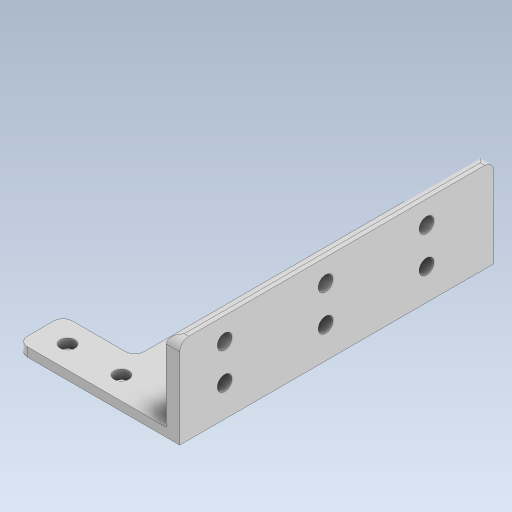
# Autodesk Inventor part: Holder Conveyor Kiri
Saved by Autodesk Inventor 2023.5 (Build 275446000, 446)
## iProperties
Created: 2025-10-12
Part Number: Holder Conveyor Kiri
Material: Generic
Document SubType Name: Modeling
Designer: Guntur
Density: 1 g/cm^3
Appearance: Default
Author: Guntur
## iProperties of the stored document Holder Conveyor Kiri_3DPrint.ipt
Created: 2025-10-20
Part Number: Holder Conveyor Kiri_3DPrint
Material: Generic
Document SubType Name: Modeling
Designer: Guntur
Density: 1 g/cm^3
Appearance: Default
Author: Guntur
Autodesk Inventor part; units mm, degrees
ref_plane "YZ Plane" through (0, 0, 0) normal (1, 0, 0) x (0, 1, 0)
ref_plane "XZ Plane" through (0, 0, 0) normal (0, 1, 0) x (-1, 0, 0)
ref_plane "XY Plane" through (0, 0, 0) normal (0, 0, 1) x (1, 0, 0)
sketch "Sketch1" plane through (0, 0, 0) normal (0, 1, 0) x (-1, 0, 0)
  circle A0 centre (0, 0) radius 1.65
  circle A1 centre (-12, 0) radius 1.65
  circle A2 centre (-20, -12.5) radius 1.65
  circle A3 centre (-20, -52.5) radius 1.65
  line L0 (-10, -30) -> (-30, -30)
  line L1 (-30, -30) -> (-30, 5)
  line L2 (-30, 5) -> (-10, 5)
  line L3 (-10, 5) -> (-10, -30)
  line L4 (-10, -30) -> (-30, 5) construction
  line L5 (-30, -30) -> (-10, 5) construction
  line L6 (-30, -5) -> (6, -5)
  line L7 (6, -5) -> (6, 5)
  line L8 (6, 5) -> (-30, 5)
  line L9 (-30, 5) -> (-30, -5)
  line L10 (-30, -5) -> (6, 5) construction
  line L11 (6, -5) -> (-30, 5) construction
  line L12 (-10, -30) -> (-30, -30)
  line L13 (-30, -30) -> (-30, -65)
  line L14 (-30, -65) -> (-10, -65)
  line L15 (-10, -65) -> (-10, -30)
  line L16 (-30, 5) -> (-27, 5)
  line L17 (-27, 5) -> (-27, -65)
  line L18 (-27, -65) -> (-30, -65)
  line L19 (-30, -65) -> (-30, 5)
  circle A4 centre (-20, -20) radius 1.65
  circle A5 centre (-20, -60) radius 1.65
  point P0 (-10, -5)
  dimension "d0" = 3.3
  dimension "d1" = 3.3
  dimension "d2" = 12
  dimension "d3" = 3.3
  dimension "d4" = 12.5
  dimension "d5" = 20
  dimension "d6" = 3.3
  dimension "d7" = 40
  dimension "d8" = 20
  dimension "d9" = 35
  dimension "d25" = 3.3
  dimension "d26" = 20
  dimension "d27" = 3.3
  dimension "d28" = 40
  constraints: 40 end point, 8 parallel, 6 centre point, 4 horizontal, 4 midpoint, 4 perpendicular, 2 point on line, 1 coincident
  measures "d0" diameter of A0
  measures "d1" diameter of A1
  measures "d2" distance of A1.centre point (0, 0)
  measures "d3" diameter of A2
  measures "d4" vertical distance of point (0, 0) A2.centre
  measures "d5" horizontal distance of point (0, 0) A2.centre
  measures "d6" diameter of A3
  measures "d7" distance of A2.centre A3.centre
  measures "d8" distance of L1.end L2.end
  measures "d9" distance of L13.end L12.end
  measures "d25" diameter of A4
  measures "d26" vertical distance of A1.centre A4.centre
  measures "d27" diameter of A5
  measures "d28" distance of A4.centre A5.centre
extrude "Extrusion1" add sketch "Sketch1" along normal blind 2 contours L15 L14 L17 L0 | L0 L17 L6 L3 | L6 L17 L2 L3 | L3 L8 L7 L6
extrude "Extrusion2" add sketch "Sketch1" along normal blind 20 contours L17 L14 L13 L0 | L0 L1 L6 L17 | L6 L1 L2 L17
sketch "Sketch2" plane through (30, 0, 5) normal (1, 0, 0) x (0, 0, -1)
  circle A0 centre (10, 15) radius 1.65
  line L0 (0, 0) -> (0, 20) projected
  circle A1 centre (55, 15) radius 1.65
  line L1 (70, 0) -> (70, 20) projected
  circle A2 centre (32.5, 15) radius 1.65
  line L2 (0, 20) -> (70, 20) projected
  line L3 (0, 2) -> (0, 20) projected
  line L4 (0, 11) -> (70, 11)
  circle A3 centre (10, 7) radius 1.65
  circle A4 centre (55, 7) radius 1.65
  circle A5 centre (32.5, 7) radius 1.65
  point P0 (5, 0)
  point P1 (70, 10)
  dimension "d14" = 3.3
  dimension "d15" = 10
  dimension "d16" = 3.3
  dimension "d18" = 3.3
  dimension "d21" = 5
  dimension "d22" = 5
  dimension "d23" = 5
  dimension "d24" = 15
  constraints: 6 centre point, 3 symmetric about line, 2 end point, 2 midpoint, 1 perpendicular, 1 point on line, 3 other
  measures "d14" diameter of A0
  measures "d15" distance from line of L0 A0.centre
  measures "d16" diameter of A1
  measures "d18" diameter of A2
  measures "d21" distance from line of L2 A0.centre
  measures "d22" distance from line of L2 A1.centre
  measures "d23" distance from line of L2 A2.centre
  measures "d24" distance from line of L1 A1.centre
extrude "Extrusion3" cut sketch "Sketch2" against normal blind 20 contours A0 | A1 | A2 | A3 | A4 | A5
fillet "Fillet1" radius 2 6 edges at (-6, 1, -5) (10, 1, -5) (27, 20, -30) (28.5, 20, 5) (28.5, 20, -65) (-6, 1, 5)
body "Solid1"
